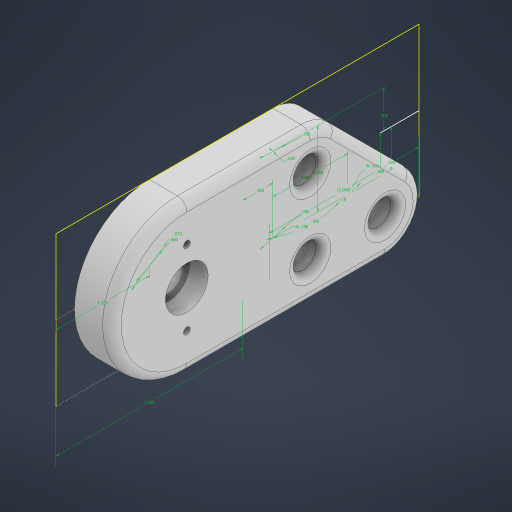
# Autodesk Inventor part: bldc_bracket
Saved by Autodesk Inventor 2024 (Build 280153000, 153)
## iProperties
Created: 2023-11-29
Part Number: bldc_bracket
Material: Generic
Document SubType Name: Modeling
Designer: jerem
Density: 1 g/cm^3
Appearance: Default
Author: jerem
## iProperties of the stored document bearing_bracket_3DPrint.ipt
Created: 2023-11-30
Part Number: bearing_bracket_3DPrint
Material: Generic
Document SubType Name: Modeling
Designer: jerem
Density: 1 g/cm^3
Appearance: Default
Author: jerem
Autodesk Inventor part; units mm, degrees
ref_plane "YZ Plane" through (0, 0, 0) normal (1, 0, 0) x (0, 1, 0)
ref_plane "XZ Plane" through (0, 0, 0) normal (0, 1, 0) x (-1, 0, 0)
ref_plane "XY Plane" through (0, 0, 0) normal (0, 0, 1) x (1, 0, 0)
sketch "Sketch1" plane through (0, 0, 0) normal (0, 1, 0) x (-1, 0, 0)
  line L0 (0, 0) -> (0, 8.89)
  line L1 (0, 0) -> (12.7, 0)
  line L2 (12.7, 0) -> (12.7, 8.89)
  line L3 (12.7, 8.89) -> (0, 8.89)
  line L4 (0, 8.89) -> (0, 72.39)
  line L5 (0, 0) -> (-139.7, 0) construction
  line L6 (12.7, 0) -> (12.7, -50.8)
  line L7 (12.7, -50.8) -> (0, -50.8)
  line L8 (0, -50.8) -> (0, 0)
  line L9 (0, 40.64) -> (-26.416, 40.64) construction
  line L10 (-26.416, 40.64) -> (-39.116, 40.64) construction
  line L11 (-39.116, 40.64) -> (-140.716, 40.64) construction
  line L12 (0, 72.39) -> (12.7, 72.39)
  line L13 (12.7, 72.39) -> (12.7, 8.89)
  dimension "d1" = 8.89
  dimension "d3" = 12.7
  dimension "d4" = 63.5
  dimension "d6" = 139.7
  dimension "d7" = 50.8
  dimension "d8" = 26.416
  dimension "d9" = 12.7
  dimension "d10" = 101.6
  dimension "d13" = 31.75
  constraints: 28 end point, 4 horizontal, 4 perpendicular, 3 vertical, 2 point on line, 1 collinear, 1 midpoint
  measures "d1" distance of L0.start L0.end
  measures "d3" distance of L0.start L1.end
  measures "d4" distance of L0.end L4.end
  measures "d6" distance of L0.start L5.end
  measures "d7" distance of L1.end L6.end
  measures "d8" distance of L9.start L9.end
  measures "d9" distance of L9.end L10.end
  measures "d10" distance of L10.end L11.end
  measures "d13" distance between parallel lines of L12 L9
extrude "Extrusion1" add sketch "Sketch1" along normal blind 50.8
sketch "Sketch2" plane through (-12.7, 0, -50.8) normal (-1, 0, 0) x (0, 0, 1)
  line L0 (123.19, 0) -> (0, 0) construction
  line L1 (0, 0) -> (50.8, 0) construction
  line L2 (50.8, 0) -> (59.69, 0) construction
  line L3 (59.69, 0) -> (123.19, 0) construction
  line L4 (123.19, 0) -> (123.19, 50.8) construction
  line L5 (0, 0) -> (0, 50.8) projected
  circle A0 centre (49.53, 38.1) radius 1.905
  circle A1 centre (24.13, 12.7) radius 1.905
  circle A2 centre (49.53, 12.7) radius 1.905
  circle A3 centre (49.53, 38.1) radius 4.445
  circle A4 centre (24.13, 12.7) radius 4.445
  circle A5 centre (49.53, 12.7) radius 4.445
  line L6 (0, 25.4) -> (13.335, 25.4)
  line L7 (59.69, 0) -> (59.69, 50.8)
  line L8 (123.19, 50.8) -> (0, 50.8) projected
  dimension "d16" = 50.8
  dimension "d17" = 63.5
  dimension "d32" = 3.81
  dimension "d34" = 3.81
  dimension "d36" = 3.81
  dimension "d38" = 8.89
  dimension "d39" = 8.89
  dimension "d40" = 8.89
  dimension "d41" = 25.4
  dimension "d42" = 25.4
  dimension "d43" = 10.16
  dimension "d49" = 12.7
  dimension "d50" = 12.7
  dimension "d51" = 12.7
  constraints: 10 end point, 6 centre point, 4 point on line, 3 coincident, 1 collinear, 1 horizontal, 1 midpoint, 1 vertical
  measures "d16" distance of L0.end L1.end
  measures "d17" distance of L2.end L3.end
  measures "d32" diameter of A0
  measures "d34" diameter of A1
  measures "d36" diameter of A2
  measures "d38" diameter of A3
  measures "d39" diameter of A4
  measures "d40" diameter of A5
  measures "d41" distance of A2.centre A0.centre
  measures "d42" distance of A2.centre A1.centre
  measures "d43" distance from line of L7 A2.centre
  measures "d49" distance from line of L6 A2.centre
  measures "d50" distance from line of L6 A1.centre
  measures "d51" distance from line of L6 A0.centre
extrude "Extrusion4" cut sketch "Sketch2" against normal through all contours A0 | A1 | A2
extrude "Extrusion5" cut sketch "Sketch2" along normal blind 7.62 from surface at -12.7 contours A0 | A3 | A4 | A5
chamfer "Chamfer1" distance 25.4 angle 45 1 edges at (-6.35, 50.8, -50.8)
fillet "Fillet3" radius 12.7 3 edges at (-6.35, 50.8, -25.4) (-6.35, 25.4, -50.8) (-6.35, 0, -50.8)
fillet "Fillet8" radius 2.54 3 edges at (0, 12.7, -31.115) (0, 12.7, -5.715) (0, 38.1, -5.715)
sketch "Sketch6" plane through (-12.7, 0, 72.39) normal (-1, 0, 0) x (0, 0, 1)
  line L0 (0, 0) -> (0, 50.8) projected
  line L1 (0, 0) -> (0, 50.8) projected
  line L2 (0, 25.4) -> (-31.75, 25.4) construction
  circle A0 centre (-31.75, 25.4) radius 7.239
  circle A1 centre (-31.75, 25.4) radius 5.08
  point P0 (-72.39, 0)
  dimension "d87" = 31.75
  dimension "d88" = 14.478
  dimension "d89" = 10.16
  constraints: 2 centre point, 2 coincident, 2 end point, 1 horizontal, 1 midpoint
  measures "d87" distance of L2.start L2.end
  measures "d88" diameter of A0
  measures "d89" diameter of A1
extrude "Extrusion11" cut sketch "Sketch6" along normal blind 6.35 from surface at -12.7
extrude "Extrusion12" cut sketch "Sketch6" against normal through all contours A1
sketch "Sketch7" plane through (-12.7, 0, 72.39) normal (-1, 0, 0) x (0, 0, 1)
  circle A0 centre (-31.75, 25.4) radius 7.239 construction
  line L0 (-31.75, 25.4) -> (-31.75, 38.1) construction
  line L1 (-31.75, 25.4) -> (-31.75, 12.7) construction
  circle A1 centre (-31.75, 38.1) radius 1.143
  circle A2 centre (-31.75, 12.7) radius 1.143
  point P0 (-72.39, 0)
  dimension "d95" = 12.7
  dimension "d96" = 12.7
  dimension "d97" = 2.286
  dimension "d98" = 2.286
  constraints: 4 end point, 2 centre point, 2 coincident, 2 vertical
  measures "d95" distance of L0.start L0.end
  measures "d96" distance of L0.start L1.end
  measures "d97" diameter of A1
  measures "d98" diameter of A2
extrude "Extrusion13" cut sketch "Sketch7" along normal blind 2.54 from surface at -12.7
sketch "Sketch8" plane through (0, 0, 72.39) normal (1, 0, 0) x (0, 0, -1)
  circle A0 centre (31.75, 25.4) radius 5.08 projected
  circle A1 centre (31.75, 25.4) radius 25.4
  line L0 (92.5295, 50.8) -> (0, 50.8) projected
  line L1 (31.75, 50.8) -> (0, 50.8)
  line L2 (0, 0) -> (0, 50.8) projected
  line L3 (0, 0) -> (31.75, 0)
  line L4 (110.49, 0) -> (0, 0) projected
  point P0 (72.39, 0)
  constraints: 4 end point, 2 point on circle, 2 point on line, 2 tangent, 1 centre point, 1 coincident, 1 collinear
extrude "Extrusion14" cut sketch "Sketch8" against normal through all contours A1 L3 L2 L0
sketch "Sketch9" plane through (-12.7, 12.7, -50.8) normal (-1, 0, 0) x (0, 0, 1)
  circle A0 centre (24.13, 0) radius 1.905 construction
  line L0 (24.13, 0) -> (24.13, -12.7) construction
  line L1 (91.44, -12.7) -> (12.7, -12.7) construction
  line L2 (24.13, 0) -> (11.43, 0) construction
  line L3 (11.43, 0) -> (11.43, 24.13)
  line L4 (21.6803, 34.3803) -> (3.7197, 16.4197) construction
  arc A1 (0, 0) -> (12.7, -12.7) centre (12.7, 0) ccw construction
  circle A2 centre (49.53, 0) radius 1.905 construction
  circle A3 centre (24.13, 0) radius 1.905 construction
  circle A4 centre (49.53, 25.4) radius 1.905 construction
  arc A5 (91.44, -12.7) -> (91.44, 38.1) centre (91.44, 12.7) ccw construction
  line L5 (30.6605, 38.1) -> (91.44, 38.1) construction
  arc A6 (30.6605, 38.1) -> (21.6803, 34.3803) centre (30.6605, 25.4) ccw construction
  line L6 (3.7197, 16.4197) -> (21.6803, 34.3803) construction
  arc A7 (3.7197, 16.4197) -> (0, 7.4395) centre (12.7, 7.4395) ccw construction
  line L7 (0, 0) -> (0, 7.4395) construction
  arc A8 (0, 0) -> (12.7, -12.7) centre (12.7, 0) ccw construction
  line L8 (12.7, -12.7) -> (91.44, -12.7) construction
  circle A9 centre (91.44, 12.7) radius 5.08 construction
  line L9 (3.7197, 16.4197) -> (21.6803, 34.3803) projected
  arc A10 (3.7197, 16.4197) -> (0, 7.4395) centre (12.7, 7.4395) ccw projected
  arc A11 (0, 0) -> (12.7, -12.7) centre (12.7, 0) ccw projected
  line L10 (0, 20.1395) -> (0, -8.6122)
  circle A12 centre (49.53, 25.4) radius 1.905 projected
  circle A13 centre (49.53, 25.4) radius 12.7
  circle A14 centre (24.13, 0) radius 6.985 projected
  circle A15 centre (24.13, 0) radius 12.7
  line L11 (15.1497, 8.9803) -> (40.5497, 34.3803)
  arc A16 (30.6605, 38.1) -> (21.6803, 34.3803) centre (30.6605, 25.4) ccw projected
  line L12 (123.19, 38.1) -> (0, 38.1) projected
  line L13 (12.7, -12.7) -> (91.44, -12.7) projected
  line L14 (24.13, -12.7) -> (12.7, -12.7)
  point P0 (50.8, -12.7)
  point P1 (11.43, -12.6363)
  point P2 (0, 7.4395)
  point P3 (49.53, 38.1)
  point P4 (24.13, -12.7)
  dimension "d108" = 12.7
  dimension "d56" = 31.75
  dimension "d57" = 2.286
  dimension "d58" = 8.89
  dimension "d59" = 2.286
  dimension "d60" = 8.89
  dimension "d61" = 2.286
  dimension "d62" = 7.62
  dimension "d63" = 2.286
  dimension "d64" = 7.62
  dimension "d65" = 6.35
  dimension "d66" = 6.35
  dimension "d67" = 6.35
  dimension "d68" = 6.35
  dimension "d69" = 6.35
  constraints: 12 end point, 3 point on circle, 2 coincident, 2 perpendicular, 2 point on line, 2 vertical, 1 centre point, 1 collinear, 1 horizontal, 1 tangent, 3 other
  measures "d108" distance of L0.start L2.end
extrude "Extrusion16" cut sketch "Sketch9" against normal through all contours A15 L13 A11 L10 A10 L9 L3 | L3 L9 A16 L12 A13 L11 A15
fillet "Fillet13" radius 3.175 6 edges at (0, 49.8333, -6.1301) (0, 50.8, 19.685) (0, 25.4, 66.04) (0, 0, 6.985) (0, 7.8399, -38.4033) (0, 34.3803, -22.9503)
fillet "Fillet14" radius 7.62 1 edges at (-12.7, 25.4, 35.56)
sketch "Sketch4" plane through (0, 0, 72.39) normal (1, 0, 0) x (0, 0, -1)
  circle A0 centre (31.75, 25.4) radius 3.175 projected
  circle A1 centre (31.75, 25.4) radius 13.97 construction
  circle A2 centre (31.75, 25.4) radius 19.05
  circle A3 centre (31.75, 25.4) radius 25.4
  line L0 (0, 0) -> (110.49, 0) projected
  line L1 (31.75, 25.4) -> (45.72, 46.6132)
  line L2 (31.75, 25.4) -> (45.72, 4.1868)
  point P0 (72.39, 0)
  point P1 (42.2275, 9.4901)
  point P2 (42.2275, 41.3099)
  dimension "d77" = 27.94
  dimension "d78" = 38.1
  constraints: 4 end point, 3 centre point, 3 coincident, 2 point on circle, 1 tangent
  measures "d77" diameter of A1
  measures "d78" diameter of A2
sketch "Sketch5" plane through (0, 0, 72.39) normal (1, 0, 0) x (0, 0, -1)
  arc A0 (31.75, 50.8) -> (31.75, 0) centre (31.75, 25.4) ccw projected
  line L0 (0, 50.8) -> (31.75, 50.8) projected
  line L1 (0, 0) -> (0, 50.8) projected
  line L2 (0, 0) -> (31.75, 0) projected
  point P0 (72.39, 0)
equation "\"d13\" = 0.5 * d4"
body "Solid1"
